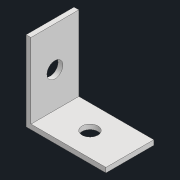
# Autodesk Inventor part: 25x25x25 Simple Angle Bracket
Saved by Autodesk Inventor 2022 (Build 260153000, 153)
## iProperties
Created: 2022-09-10
Part Number: 25x25x25 Simple Angle Bracket
Material: Generic
Document SubType Name: Modeling
Designer: robpl
Density: 1 g/cm^3
Appearance: Default
Author: robpl
Autodesk Inventor part; units mm, degrees
ref_plane "YZ Plane" through (0, 0, 0) normal (1, 0, 0) x (0, 1, 0)
ref_plane "XZ Plane" through (0, 0, 0) normal (0, 1, 0) x (-1, 0, 0)
ref_plane "XY Plane" through (0, 0, 0) normal (0, 0, 1) x (1, 0, 0)
sketch "Sketch1" plane through (0, 0, 0) normal (0, 0, 1) x (1, 0, 0)
  line L0 (0, 0) -> (25, 0)
  line L1 (25, 0) -> (25, 1.5)
  line L2 (25, 1.5) -> (0, 1.5)
  line L3 (0, 1.5) -> (0, 0)
  line L4 (0, 1.5) -> (1.5, 1.5)
  line L5 (1.5, 1.5) -> (1.5, 25)
  line L6 (1.5, 25) -> (0, 25)
  line L7 (0, 25) -> (0, 1.5)
  point P0 (1.5, 1.5)
  dimension "d0" = 25
  dimension "d1" = 1.5
  dimension "d2" = 25
  constraints: 16 end point, 4 parallel, 3 perpendicular, 2 horizontal
  measures "d0" distance of L2.end L1.end
  measures "d1" distance of L1.end L0.end
  measures "d2" distance between parallel lines of L0 L6
extrude "Extrusion1" add sketch "Sketch1" along normal blind 15
sketch "Sketch2" plane through (0, 0, 0) normal (0, -1, 0) x (1, 0, 0)
  point P0 (0, 0)
  point P1 (12.5, 7.5)
  dimension "d5" = 12.5
  dimension "d6" = 7.5
  measures "d5" horizontal distance of point (12.5, 7.5) point (0, 0)
  measures "d6" vertical distance of point (0, 0) point (12.5, 7.5)
hole "Hole1" at (12.5, 0, 7.5) direction (0, 1, 0) diameter 5 depth 8 tip angle 118
sketch "Sketch3" plane through (0, 0, 0) normal (-1, 0, 0) x (0, 0, 1)
  point P0 (0, 0)
  point P1 (7.5, 12.5)
  dimension "d14" = 12.5
  dimension "d15" = 7.5
  measures "d14" vertical distance of point (0, 0) point (7.5, 12.5)
  measures "d15" horizontal distance of point (7.5, 12.5) point (0, 0)
hole "Hole2" at (0, 12.5, 7.5) direction (1, 0, 0) diameter 5 depth 8 tip angle 118
equation "\"d2\" = d0"
body "Solid1"
